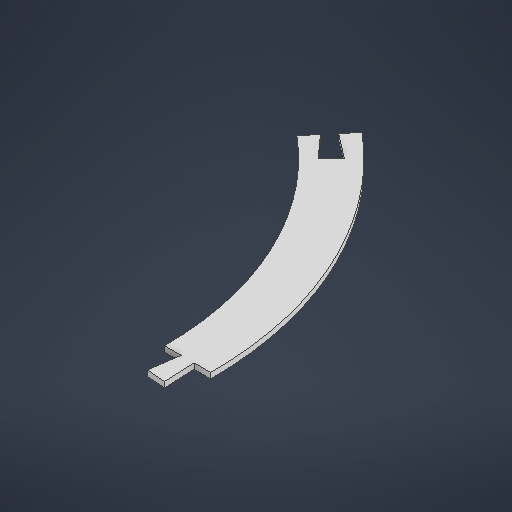
# Autodesk Inventor part: base
Saved by Autodesk Inventor 2026.2 (Build 302298000, 298)
## iProperties
Created: 2026-02-13
Part Number: base
Material: Genérico
Document SubType Name: Chapa de metal
Designer: Ian
Density: 1 g/cm^3
Appearance: Padrão
Sheet Metal Rule: Padrão
Author: Ian
Autodesk Inventor part; units mm, degrees
ref_plane "YZ Plane" through (0, 0, 0) normal (1, 0, 0) x (0, 1, 0)
ref_plane "XZ Plane" through (0, 0, 0) normal (0, 1, 0) x (-1, 0, 0)
ref_plane "XY Plane" through (0, 0, 0) normal (0, 0, 1) x (1, 0, 0)
sketch "Esboço1" plane through (0, 0, 0) normal (0, 1, 0) x (-1, 0, 0)
  arc A0 (-350, 0) -> (-247.4874, -247.4874) centre (0, 0) ccw
  arc A1 (-400, 0) -> (-282.8427, -282.8427) centre (0, 0) ccw
  circle A2 centre (0, 0) radius 400
  circle A3 centre (0, 0) radius 350
  line L0 (0, 0) -> (-407.9373, -407.9373)
  line L1 (0, 0) -> (-1224.3013, 0) construction
  line L2 (-350, 0) -> (-400, 0)
  point P0 (-282.8427, -282.8427)
  point P1 (-247.4874, -247.4874)
  dimension "d27" = 700
  dimension "d28" = 800
  dimension "d87" = 45
  constraints: 6 end point, 6 point on circle, 4 coincident, 3 centre point, 1 horizontal, 1 horizontal alignment, 3 other
  measures "d27" diameter of A0
  measures "d28" diameter of A1
  measures "d87" angle of L1 L0
extrude "Extrusão1" add sketch "Esboço1" along normal blind 6 contours A0 L0 A1 L2
sketch "Esboço5" plane through (0, 6, 0) normal (0, 1, 0) x (1, 0, 0)
  arc A0 (400, 0) -> (282.8427, 282.8427) centre (0, 0) ccw projected
  circle A1 centre (0, 0) radius 400
  circle A2 centre (0, 0) radius 350
  line L0 (0, 0) -> (299.5408, 356.9788)
  line L1 (282.8427, 282.8427) -> (247.4874, 247.4874) projected
  line L2 (282.8427, 282.8427) -> (272.2361, 272.2361)
  line L3 (272.2361, 272.2361) -> (258.094, 258.094)
  line L4 (258.094, 258.094) -> (247.4874, 247.4874)
  line L5 (257.115, 306.4178) -> (245.5449, 292.629)
  line L6 (245.5449, 292.629) -> (236.5458, 281.9044)
  line L7 (236.5458, 281.9044) -> (224.9757, 268.1156)
  line L8 (258.094, 258.094) -> (236.5458, 281.9044)
  line L9 (272.2361, 272.2361) -> (245.5449, 292.629)
  dimension "d88" = 5
  dimension "d89" = 15
  dimension "d90" = 20
  dimension "d91" = 18
  dimension "d92" = 14
  constraints: 18 end point, 6 point on line, 2 coincident, 1 centre point, 1 collinear, 1 point on circle, 4 other
  measures "d88" angle of L1 L0
  measures "d89" distance of L1.start L2.end
  measures "d90" distance of L2.end L3.end
  measures "d91" distance of L5.start L5.end
  measures "d92" distance of L5.end L6.end
extrude "Extrusão5" add sketch "Esboço5" against normal up to surface (6 mm away) contours L1 L9 L0 A1 | L1 A2 L0 L8
sketch "Esboço6" plane through (0, 6, 0) normal (0, 1, 0) x (1, 0, 0)
  arc A0 (400, 0) -> (257.115, 306.4178) centre (0, 0) ccw projected
  circle A1 centre (0, 0) radius 400
  arc A2 (350, 0) -> (224.9757, 268.1156) centre (0, 0) ccw projected
  circle A3 centre (0, 0) radius 350
  line L0 (0, 0) -> (512.6153, -44.848)
  line L1 (350, 0) -> (400, 0) projected
  line L2 (350, 0) -> (368, 0)
  line L3 (368, 0) -> (382, 0)
  line L4 (382, 0) -> (400, 0)
  line L5 (348.6681, -30.5045) -> (363.6111, -31.8118)
  line L6 (363.6111, -31.8118) -> (383.535, -33.555)
  line L7 (383.535, -33.555) -> (398.4779, -34.8623)
  line L8 (368, 0) -> (363.6111, -31.8118)
  line L9 (382, 0) -> (383.535, -33.555)
  dimension "d93" = 5
  dimension "d94" = 18
  dimension "d95" = 14
  dimension "d96" = 15
  dimension "d97" = 20
  constraints: 18 end point, 6 point on line, 4 point on circle, 2 centre point, 2 coincident, 1 collinear
  measures "d93" angle of L1 L0
  measures "d94" distance of L1.start L2.end
  measures "d95" distance of L2.end L3.end
  measures "d96" distance of L5.start L5.end
  measures "d97" distance of L5.end L6.end
extrude "Extrusão6" add sketch "Esboço6" against normal up to surface (6 mm away) contours L9 L0 L8 L1
